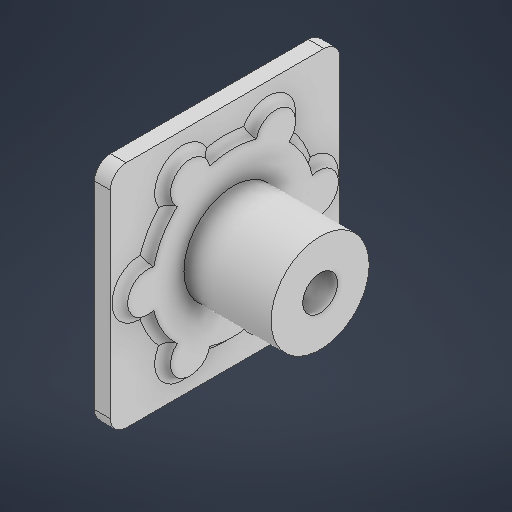
# Autodesk Inventor part: BASE COVER (actual)
Saved by Autodesk Inventor 2025.2 (Build 292293000, 293)
## iProperties
Created: 2025-10-07
Part Number: BASE COVER (actual)
Material: Generic
Document SubType Name: Modeling
Designer: elaij
Density: 1 g/cm^3
Appearance: Default
Author: elaij
Autodesk Inventor part; units mm, degrees
ref_plane "YZ Plane" through (0, 0, 0) normal (1, 0, 0) x (0, 1, 0)
ref_plane "XZ Plane" through (0, 0, 0) normal (0, 1, 0) x (-1, 0, 0)
ref_plane "XY Plane" through (0, 0, 0) normal (0, 0, 1) x (1, 0, 0)
sketch "Sketch2" plane through (0, 0, 0) normal (1, 0, 0) x (0, 1, 0)
  line L0 (0, 0) -> (46.7654, -27)
  circle A0 centre (46.7654, -27) radius 12.5
  circle A1 centre (46.7654, 27) radius 12.5
  circle A2 centre (0, 54) radius 12.5
  circle A3 centre (-46.7654, 27) radius 12.5
  circle A4 centre (-46.7654, -27) radius 12.5
  circle A5 centre (0, -54) radius 12.5
  line L1 (0, 0) -> (12.8411, 0)
  arc A6 (49.3373, -14.7675) -> (49.3373, 14.7675) centre (0, 0) ccw
  arc A7 (51.7204, -15.5241) -> (51.7204, 15.5241) centre (0, 0) ccw
  arc A8 (12.416, -52.5532) -> (46.7654, -27) centre (0, 0) ccw
  arc A9 (11.8797, -50.1111) -> (37.4577, -35.3437) centre (0, 0) ccw
  arc A10 (-39.3044, -37.0292) -> (-12.416, -52.5532) centre (0, 0) ccw
  arc A11 (-37.4577, -35.3437) -> (-11.8797, -50.1111) centre (0, 0) ccw
  arc A12 (-51.7204, 15.5241) -> (-51.7204, -15.5241) centre (0, 0) ccw
  arc A13 (-49.3373, 14.7675) -> (-49.3373, -14.7675) centre (0, 0) ccw
  arc A14 (37.4577, 35.3437) -> (11.8797, 50.1111) centre (0, 0) ccw
  arc A15 (-11.8797, 50.1111) -> (-37.4577, 35.3437) centre (0, 0) ccw
  arc A16 (39.3044, 37.0292) -> (12.416, 52.5532) centre (0, 0) ccw
  arc A17 (-12.416, 52.5532) -> (-39.3044, 37.0292) centre (0, 0) ccw
  dimension "d11" = 360
  dimension "d13" = 30
  dimension "d15" = 25
  constraints: 47 point on circle, 18 centre point, 4 end point, 3 coincident, 1 horizontal, 13 other
  measures "d13" angle of L1 L0
  measures "d15" diameter of A0
extrude "Extrusion2" add sketch "Sketch2" against normal blind 5 contours A0 A8 L0 | A0 A9 A5 A11 A4 A13 A3 A15 A2 A14 A1 A6 | L0 A8 A0 | A1 | A5 | A2 | A4 | A3
sketch "Sketch5" plane through (-5, 0, 0) normal (-1, 0, 0) x (0, 0, 1)
  line L0 (-62.5, 62.5) -> (62.5, 62.5)
  line L1 (62.5, 62.5) -> (62.5, -62.5)
  line L2 (62.5, -62.5) -> (-62.5, -62.5)
  line L3 (-62.5, -62.5) -> (-62.5, 62.5)
  circle A0 centre (62.5, 62.5) radius 10
  circle A1 centre (62.5, -62.5) radius 10
  circle A2 centre (-62.5, 62.5) radius 10
  circle A3 centre (-62.5, -62.5) radius 10
  line L4 (-72.5, 72.5) -> (72.5, 72.5)
  line L5 (72.5, 72.5) -> (72.5, -72.5)
  line L6 (72.5, -72.5) -> (-72.5, -72.5)
  line L7 (-72.5, -72.5) -> (-72.5, 72.5)
  point P0 (0, 0)
  point P1 (62.5, 72.5)
  point P2 (-62.5, 72.5)
  point P3 (-72.5, 62.5)
  point P4 (-72.5, -62.5)
  point P5 (-62.5, -72.5)
  point P6 (62.5, -72.5)
  point P7 (72.5, -62.5)
  point P8 (72.5, 62.5)
  dimension "d40" = 125
  dimension "d41" = 62.5
  dimension "d42" = 125
  dimension "d43" = 62.5
  dimension "d46" = 125
  dimension "d49" = 125
  dimension "d52" = 20
  constraints: 16 end point, 4 centre point, 4 parallel, 4 tangent, 3 horizontal, 2 perpendicular, 1 coincident, 1 vertical, 6 other
  measures "d40" distance between parallel lines of L1 L3
  measures "d41" distance from line of point (0, 0) L1
  measures "d42" distance between parallel lines of L2 L0
  measures "d43" distance from line of point (0, 0) L2
  measures "d46" distance of A0.centre A1.centre
  measures "d49" distance of A0.centre A2.centre
  measures "d52" diameter of A0
extrude "Extrusion5" add sketch "Sketch5" along normal blind 10 contours L3 A2 L0 | L0 A2 L3 | A2 L4 A0 L0 | L0 A0 L1 A1 L2 A3 L3 A2 | L3 A3 L7 A2 | A0 L1 L0 | L0 L1 A0 | A3 L2 L3 | L3 L2 A3 | A0 L5 A1 L1 | L2 A1 L6 A3 | A1 L2 L1 | L1 L2 A1
sketch "Sketch6" plane through (-15, 0, 0) normal (-1, 0, 0) x (0, 0, 1)
  line L0 (-62.5, 62.5) -> (62.5, 62.5)
  line L1 (62.5, 62.5) -> (62.5, -62.5)
  line L2 (62.5, -62.5) -> (-62.5, -62.5)
  line L3 (-62.5, -62.5) -> (-62.5, 62.5)
  circle A0 centre (62.5, 62.5) radius 10
  circle A1 centre (62.5, -62.5) radius 10
  circle A2 centre (-62.5, 62.5) radius 10
  circle A3 centre (-62.5, -62.5) radius 10
  line L4 (-72.5, 72.5) -> (72.5, 72.5)
  line L5 (72.5, 72.5) -> (72.5, -72.5)
  line L6 (72.5, -72.5) -> (-72.5, -72.5)
  line L7 (-72.5, -72.5) -> (-72.5, 72.5)
  point P0 (0, 0)
  point P1 (0, 0)
  point P2 (91.0413, 95.2532)
  point P3 (-33.9587, 95.2532)
  point P4 (-43.9587, 85.2532)
  point P5 (-43.9587, -39.7468)
  point P6 (-33.9587, -49.7468)
  point P7 (91.0413, -49.7468)
  point P8 (101.0413, -39.7468)
  point P9 (101.0413, 85.2532)
  point P10 (-62.5, -52.5)
  point P11 (-52.5, -62.5)
  point P12 (52.5, -62.5)
  point P13 (62.5, -52.5)
  point P14 (62.5, 52.5)
  point P15 (52.5, 62.5)
  point P16 (-52.5, 62.5)
  point P17 (-62.5, 52.5)
  dimension "d59" = 125
  dimension "d60" = 62.5
  dimension "d61" = 125
  dimension "d62" = 62.5
  dimension "d63" = 125
  dimension "d64" = 125
  dimension "d65" = 20
  dimension "d66" = 0
  dimension "d67" = 0
  constraints: 16 end point, 4 centre point, 4 parallel, 4 tangent, 3 horizontal, 2 perpendicular, 1 coincident, 1 vertical, 6 other
  measures "d59" distance between parallel lines of L1 L3
  measures "d60" distance from line of point (0, 0) L1
  measures "d61" distance between parallel lines of L2 L0
  measures "d62" distance from line of point (0, 0) L2
  measures "d63" distance of A0.centre A1.centre
  measures "d64" distance of A0.centre A2.centre
  measures "d65" diameter of A0
  measures "d66" distance of point (0, 0) point (0, 0)
  measures "d67" distance of point (0, 0) point (0, 0)
extrude "Extrusion6" cut sketch "Sketch6" against normal blind 4 contours L0 A0 L1 A1 L2 A3 L3 A2
sketch "Sketch7" plane through (-11, 0, 0) normal (-1, 0, 0) x (0, 0, 1)
  circle A0 centre (0, 0) radius 37.5
  dimension "d70" = 75
  constraints: 1 centre point, 1 coincident
  measures "d70" diameter of A0
extrude "Extrusion7" add sketch "Sketch7" along normal blind 15
sketch "Sketch8" plane through (0, 0, 0) normal (1, 0, 0) x (0, 0, -1)
  circle A0 centre (0, 0) radius 31
  dimension "d73" = 62
  constraints: 1 centre point, 1 coincident
  measures "d73" diameter of A0
extrude "Extrusion8" add sketch "Sketch8" along normal blind 55
sketch "Sketch9" plane through (-26, 0, 0) normal (-1, 0, 0) x (0, 0, 1)
  point P0 (0, 0)
  point P1 (0, 0)
  constraints: 1 coincident
hole "Hole1" at (-26, 0, 0) direction (1, 0, 0) diameter 22 end through all
fillet "Fillet2" radius 5 12 edges at (-5, 57.5907, -33.25) (-5, 25.75, -44.6003) (-5, 0, -66.5) (-5, -25.75, -44.6003) (-5, -57.5907, -33.25) (-5, -51.5, 0) (-5, -57.5907, 33.25) (-5, -25.75, 44.6003) (-5, 0, 66.5) (-5, 25.75, 44.6003) (-5, 57.5907, 33.25) (-5, 51.5, 0)
body "Solid2"
